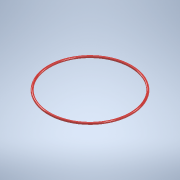
# Autodesk Inventor part: Sello Plato Oring2155
Saved by Autodesk Inventor 2020 (Build 240168000, 168)
## iProperties
Created: 2020-06-08
Part Number: Sello Plato Oring2155
Material: Rubber, Silicone
Document SubType Name: Modeling
Designer: Bruno
Density: 1.25 g/cm^3
Appearance: Orange-Red
Author: Bruno
Autodesk Inventor part; units mm, degrees
ref_plane "YZ Plane" through (0, 0, 0) normal (1, 0, 0) x (0, 1, 0)
ref_plane "XY Plane" through (0, 0, 0) normal (0, 0, 1) x (1, 0, 0)
sketch "Sketch1" plane through (0, 0, 0) normal (0, 0, 1) x (1, 0, 0)
  circle A0 centre (-48.77, 0) radius 1.31
  line L0 (0, 0) -> (0, 34.5509)
  dimension "d0" = 2.62
  dimension "d2" = 48.77
  constraints: 2 end point, 1 centre point, 1 vertical
  measures "d0" diameter of A0
  measures "d2" distance of L0.start A0.centre
revolve "Revolution1" add sketch "Sketch1" angle 360 about axis through (0, 0, 0) along (0, 1, 0)
sketch "Sketch2" plane through (0, 0, 0) normal (0, 1, 0) x (-1, 0, 0)
  circle A0 centre (0, 0) radius 52.7902
  constraints: 1 centre point, 1 coincident
ref_plane "Work Plane1" through (0, -1.31, 0) normal (0, 1, 0) x (-1, 0, 0)
sketch "Sketch4" plane through (0, -1.31, 0) normal (0, 1, 0) x (-1, 0, 0)
  circle A0 centre (0, 0) radius 50.5
  dimension "d5" = 101
  constraints: 1 centre point, 1 coincident
  measures "d5" diameter of A0
ref_plane "Work Plane2" through (0, 1.31, 0) normal (0, 1, 0) x (-1, 0, 0)
sketch "Sketch5" plane through (0, 1.31, 0) normal (0, 1, 0) x (-1, 0, 0)
  circle A0 centre (0, 0) radius 48.4376
  constraints: 1 centre point, 1 coincident
body "Solid1"
